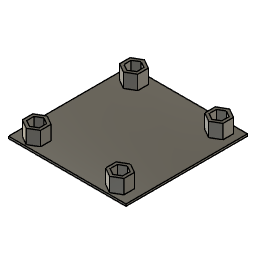
u2d2 port v2 (Autodesk Fusion 360 design; units mm, degrees)
Autodesk Fusion 360 part; units mm, degrees
sketch "Sketch1" plane through (0, 0, 0) normal (0, 0, 1) x (1, 0, 0)
  line L0 (0, 0) -> (67, 0)
  line L1 (67, 0) -> (67, 60)
  line L2 (67, 60) -> (0, 60)
  line L3 (0, 60) -> (0, 0)
  dimension "d1" = 67
  dimension "d2" = 60
  constraint horizontal L0
  constraint vertical L1
  constraint horizontal L2
  constraint vertical L3
  constraint coincident L0.start L3.end
  measures "d1" distance of L0.start L0.end
  measures "d2" distance of L0.start L2.end
extrude "Extrude1" add sketch "Sketch1" along normal blind 1 makes body 1
sketch "Sketch2" plane through (0, 0, 1) normal (0, 0, 1) x (-1, 0, 0)
  line L0 (0, -60) -> (0, 0)
  line L1 (0, 0) -> (-67, 0)
  line L2 (-67, 0) -> (-67, -60)
  line L3 (-67, -60) -> (0, -60)
  line L4 (-57, -60) -> (-57, 0)
  line L5 (-10.9779, -55.8771) -> (-7.8284, -57.5781)
  line L6 (-7.8284, -57.5781) -> (-4.7804, -55.701)
  line L7 (-4.7804, -55.701) -> (-4.8821, -52.1229)
  line L8 (-4.8821, -52.1229) -> (-8.0316, -50.4219)
  line L9 (-8.0316, -50.4219) -> (-11.0796, -52.299)
  line L10 (-11.0796, -52.299) -> (-10.9779, -55.8771)
  line L11 (-12.43, -56.5981) -> (-7.93, -59.1962)
  line L12 (-7.93, -59.1962) -> (-3.43, -56.5981)
  line L13 (-3.43, -56.5981) -> (-3.43, -51.4019)
  line L14 (-3.43, -51.4019) -> (-7.93, -48.8038)
  line L15 (-7.93, -48.8038) -> (-12.43, -51.4019)
  line L16 (-12.43, -51.4019) -> (-12.43, -56.5981)
  line L17 (-53.1, -55.7898) -> (-50, -57.5796)
  line L18 (-50, -57.5796) -> (-46.9, -55.7898)
  line L19 (-46.9, -55.7898) -> (-46.9, -52.2102)
  line L20 (-46.9, -52.2102) -> (-50, -50.4204)
  line L21 (-50, -50.4204) -> (-53.1, -52.2102)
  line L22 (-53.1, -52.2102) -> (-53.1, -55.7898)
  line L23 (-54.4959, -56.6052) -> (-49.9918, -59.1961)
  line L24 (-49.9918, -59.1961) -> (-45.4959, -56.5909)
  line L25 (-45.4959, -56.5909) -> (-45.5041, -51.3948)
  line L26 (-45.5041, -51.3948) -> (-50.0082, -48.8039)
  line L27 (-50.0082, -48.8039) -> (-54.5041, -51.4091)
  line L28 (-54.5041, -51.4091) -> (-54.4959, -56.6052)
  line L29 (-11.03, -7.7498) -> (-7.93, -9.5396)
  line L30 (-7.93, -9.5396) -> (-4.83, -7.7498)
  line L31 (-4.83, -7.7498) -> (-4.83, -4.1702)
  line L32 (-4.83, -4.1702) -> (-7.93, -2.3804)
  line L33 (-7.93, -2.3804) -> (-11.03, -4.1702)
  line L34 (-11.03, -4.1702) -> (-11.03, -7.7498)
  line L35 (-12.43, -8.5581) -> (-7.93, -11.1562)
  line L36 (-7.93, -11.1562) -> (-3.43, -8.5581)
  line L37 (-3.43, -8.5581) -> (-3.43, -3.3619)
  line L38 (-3.43, -3.3619) -> (-7.93, -0.7638)
  line L39 (-7.93, -0.7638) -> (-12.43, -3.3619)
  line L40 (-12.43, -3.3619) -> (-12.43, -8.5581)
  line L41 (-52.17, -7.7898) -> (-49.07, -9.5796)
  line L42 (-49.07, -9.5796) -> (-45.97, -7.7898)
  line L43 (-45.97, -7.7898) -> (-45.97, -4.2102)
  line L44 (-45.97, -4.2102) -> (-49.07, -2.4204)
  line L45 (-49.07, -2.4204) -> (-52.17, -4.2102)
  line L46 (-52.17, -4.2102) -> (-52.17, -7.7898)
  line L47 (-53.57, -8.5981) -> (-49.07, -11.1962)
  line L48 (-49.07, -11.1962) -> (-44.57, -8.5981)
  line L49 (-44.57, -8.5981) -> (-44.57, -3.4019)
  line L50 (-44.57, -3.4019) -> (-49.07, -0.8038)
  line L51 (-49.07, -0.8038) -> (-53.57, -3.4019)
  line L52 (-53.57, -3.4019) -> (-53.57, -8.5981)
  point P0 (-7.93, -5.96)
  point P1 (-7.93, -54)
  point P2 (-50, -54)
  point P3 (-49.07, -6)
  point P4 (-7.93, -54)
  point P5 (-7.93, -54)
  point P6 (-50, -54)
  point P7 (-50, -54)
  point P8 (-7.93, -5.96)
  point P9 (-7.93, -5.96)
  point P10 (-49.07, -6)
  point P11 (-49.07, -6)
  dimension "d5" = 48.04
  dimension "d7" = 42.07
  dimension "d8" = 7
  dimension "d9" = 6
  dimension "d10" = 3.1
  dimension "d11" = 4.5
  dimension "d12" = 3.1
  dimension "d13" = 4.5
  dimension "d14" = 3.1
  dimension "d15" = 4.5
  dimension "d16" = 3.1
  dimension "d17" = 4.5
  constraint coincident L3 L4.start
  constraint coincident L1 L4.end
  constraint perpendicular L1 L4
  constraint coincident P5 P4
  constraint coincident P6 P2
  constraint coincident P7 P6
  constraint coincident P9 P8
  constraint coincident P11 P10
  measures "d5" distance of P9 P4
  measures "d7" distance of P5 P2
  measures "d8" distance of P6 L4
  measures "d9" distance of L3 P5
  measures "d10" distance of P5 L10
  measures "d11" distance of P5 L16
  measures "d12" distance of P7 L22
  measures "d13" distance of P7 L28
  measures "d14" distance of P9 L34
  measures "d15" distance of P9 L40
  measures "d16" distance of P11 L46
  measures "d17" distance of P11 L52
extrude "Extrude2" add sketch "Sketch2" along normal blind 7 contours L11 L12 L13 L14 L15 L16 | L23 L24 L25 L26 L27 L28 | L35 L36 L37 L38 L39 L40 | L47 L48 L49 L50 L51 L52 bodies 1
extrude "Extrude3" cut 1 faces at (67, 20, 0.3333) along direction (-1, 0, 0) blind 9 on bodies 1 bodies 1
extrude "Extrude4" add 4 faces at (8.9799, 53.433, 1) (51.0333, 53.4034, 1) (48.0367, 5.4034, 1) (8.9633, 6.5566, 1) along direction (0, 0, 1) blind 1 on bodies 1 bodies 1
copy_body "Body->Comp1" bodies 1 removing the originals makes body 2 in component "Component"
component "Component" placed x (1, 0, 0) y (0, 1, 0) z (0, 0, 1) at (0, 0, 0)
